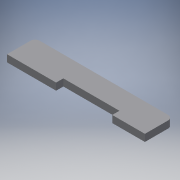
# Autodesk Inventor part: shovel_support
Saved by Autodesk Inventor 2017 (Build 210142000, 142)
## iProperties
Created: 2017-11-11
Part Number: shovel_support
Material: Generic
Document SubType Name: Modeling
Designer: Nic
Density: 1 g/cm^3
Appearance: Default
Author: Nic
Autodesk Inventor part; units mm, degrees
ref_plane "YZ Plane" through (0, 0, 0) normal (1, 0, 0) x (0, 1, 0)
ref_plane "XZ Plane" through (0, 0, 0) normal (0, 1, 0) x (-1, 0, 0)
ref_plane "XY Plane" through (0, 0, 0) normal (0, 0, 1) x (1, 0, 0)
sketch "Sketch1" plane through (0, 0, 0) normal (0, 0, 1) x (1, 0, 0)
  line L0 (-35, 0) -> (-35, 12)
  line L1 (-35, 12) -> (24, 12)
  line L2 (24, 12) -> (24, 0)
  line L3 (24, 0) -> (10, 0)
  line L4 (10, 0) -> (10, 3.1)
  line L5 (10, 3.1) -> (-14, 3.1)
  line L6 (-14, 3.1) -> (-14, 0)
  line L7 (-14, 0) -> (-35, 0)
  line L8 (0, 0) -> (0, 12) construction
  line L9 (-14, 0) -> (0, 0) construction
  dimension "d0" = 3.1
  dimension "d1" = 24
  dimension "d3" = 12
  dimension "d7" = 10
  dimension "d8" = 24
  dimension "d9" = 35
  constraints: 20 end point, 8 perpendicular, 2 point on line, 1 horizontal, 1 vertical
  measures "d0" distance between parallel lines of L5 L3
  measures "d1" distance of L4.end L5.end
  measures "d3" distance of L1.end L2.end
  measures "d7" distance between parallel lines of L4 L8
  measures "d8" distance between parallel lines of L2 L8
  measures "d9" distance between parallel lines of L0 L8
extrude "Extrusion1" add sketch "Sketch1" along normal blind 3
fillet "Fillet1" radius 2 2 edges at (-35, 12, 1.5) (24, 12, 1.5)
body "Solid1"
